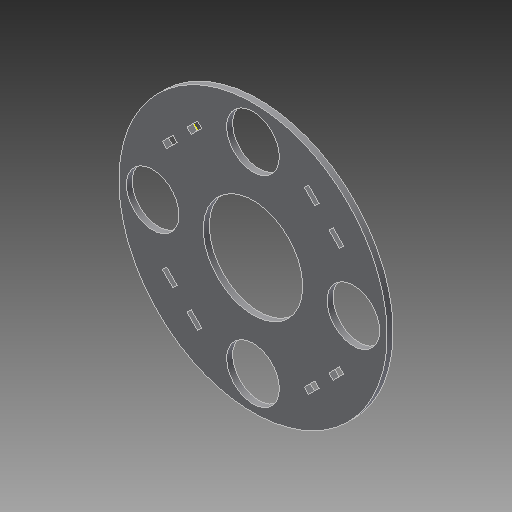
# Autodesk Inventor part: Диск_верхний_В5
Saved by Autodesk Inventor 2021.3 (Build 253353000, 353)
## iProperties
RuleStatus: InUse
Part Number: Диск_верхний_В5
Checked By: Якушев
Engr Approved By: Малов
Material: По умолчанию1
Document SubType Name: Modeling
Mfg Approved By: Судаков
Designer: Смирнов
Density: 1 g/cm^3
Appearance: По умолчанию1
AfterMaterialChange0: Материал
BeforeDocSave0: Материал
AfterAnyiPropertyChange0: Материал
Материал: По умолчанию1
Author: Смирнов
Autodesk Inventor part; units mm, degrees
ref_plane "YZ Plane" through (0, 0, 0) normal (1, 0, 0) x (0, 1, 0)
ref_plane "XZ Plane" through (0, 0, 0) normal (0, 1, 0) x (-1, 0, 0)
ref_plane "XY Plane" through (0, 0, 0) normal (0, 0, 1) x (1, 0, 0)
ref_plane "РабПлоскость1" through (-64.3467, 78.4889, 38) normal (0, 0, 1) x (-0.7071, -0.7071, 0)
sketch "Эскиз1" plane through (-64.3467, 78.4889, 38) normal (0, 0, 1) x (-0.7071, -0.7071, 0)
  circle A0 centre (10, 101) radius 135 projected
  line L0 (35, 205) -> (35, 199) projected
  line L1 (35, 199) -> (20, 199) projected
  line L2 (20, 199) -> (20, 205) projected
  line L3 (20, 205) -> (35, 205) projected
  line L4 (-15, 205) -> (0, 205) projected
  line L5 (0, 205) -> (0, 199) projected
  line L6 (0, 199) -> (-15, 199) projected
  line L7 (-15, 199) -> (-15, 205) projected
  line L8 (114, 76) -> (108, 76) projected
  line L9 (108, 76) -> (108, 91) projected
  line L10 (108, 91) -> (114, 91) projected
  line L11 (114, 91) -> (114, 76) projected
  line L12 (114, 126) -> (114, 111) projected
  line L13 (114, 111) -> (108, 111) projected
  line L14 (108, 111) -> (108, 126) projected
  line L15 (108, 126) -> (114, 126) projected
  line L16 (-15, -3) -> (-15, 3) projected
  line L17 (-15, 3) -> (0, 3) projected
  line L18 (0, 3) -> (0, -3) projected
  line L19 (0, -3) -> (-15, -3) projected
  line L20 (35, -3) -> (20, -3) projected
  line L21 (20, -3) -> (20, 3) projected
  line L22 (20, 3) -> (35, 3) projected
  line L23 (35, 3) -> (35, -3) projected
  line L24 (-88, 111) -> (-94, 111) projected
  line L25 (-94, 111) -> (-94, 126) projected
  line L26 (-94, 126) -> (-88, 126) projected
  line L27 (-88, 126) -> (-88, 111) projected
  line L28 (-94, 91) -> (-88, 91) projected
  line L29 (-88, 91) -> (-88, 76) projected
  line L30 (-88, 76) -> (-94, 76) projected
  line L31 (-94, 76) -> (-94, 91) projected
  circle A1 centre (10, 101) radius 50 projected
  circle A2 centre (10, 101) radius 135 projected
  circle A3 centre (81.4178, 29.5822) radius 26.5 projected
  circle A4 centre (-61.4178, 29.5822) radius 26.5 projected
  circle A5 centre (-61.4178, 172.4178) radius 26.5 projected
  circle A6 centre (81.4178, 172.4178) radius 26.5 projected
  point P0 (10, 101)
extrude "Выдавливание1" add sketch "Эскиз1" along normal blind 6
